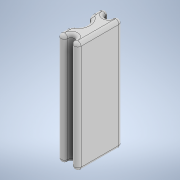
# Autodesk Inventor part: CableBase
Saved by Autodesk Inventor 2020 (Build 240168000, 168)
## iProperties
Created: 2020-07-28
Part Number: CableBase
Material: Generic
Document SubType Name: Modeling
Designer: maple
Density: 1 g/cm^3
Appearance: Default
Author: maple
Autodesk Inventor part; units mm, degrees
ref_plane "YZ Plane" through (0, 0, 0) normal (1, 0, 0) x (0, 1, 0)
ref_plane "XZ Plane" through (0, 0, 0) normal (0, 1, 0) x (-1, 0, 0)
ref_plane "XY Plane" through (0, 0, 0) normal (0, 0, 1) x (1, 0, 0)
sketch "Sketch1" plane through (0, 0, 0) normal (0, 1, 0) x (-1, 0, 0)
  line L0 (0, 0) -> (3, 0)
  line L1 (3, 0) -> (3, -20)
  line L2 (3, -20) -> (0, -20)
  line L3 (0, -20) -> (0, 0)
  line L4 (3, 0) -> (6, 0)
  line L5 (6, 0) -> (6, -3)
  line L6 (6, -3) -> (3, -3)
  line L7 (3, -3) -> (3, 0)
  line L8 (3, -20) -> (6, -20)
  line L9 (6, -20) -> (6, -17)
  line L10 (6, -17) -> (3, -17)
  line L11 (3, -17) -> (3, -20)
  line L12 (3, -3) -> (9, -3)
  line L13 (9, -3) -> (9, -6)
  line L14 (9, -6) -> (3, -6)
  line L15 (3, -6) -> (3, -3)
  line L16 (3, -17) -> (9, -17)
  line L17 (9, -17) -> (9, -14)
  line L18 (9, -14) -> (3, -14)
  line L19 (3, -14) -> (3, -17)
  line L20 (9, -17) -> (6, -17)
  line L21 (6, -17) -> (6, -20)
  line L22 (6, -20) -> (9, -20)
  line L23 (9, -20) -> (9, -17)
  line L24 (9, -3) -> (6, -3)
  line L25 (6, -3) -> (6, 0)
  line L26 (6, 0) -> (9, 0)
  line L27 (9, 0) -> (9, -3)
  line L28 (6, -6) -> (6, -17)
  arc A0 (9, -6) -> (9, -14) centre (10.1667, -10) ccw
  dimension "d0" = 3
  dimension "d1" = 20
  dimension "d2" = 3
  dimension "d3" = 3
  dimension "d4" = 3
  dimension "d5" = 3
  dimension "d6" = 6
  dimension "d7" = 3
  dimension "d8" = 6
  dimension "d9" = 3
  constraints: 58 end point, 14 parallel, 7 horizontal, 7 perpendicular, 2 point on circle, 1 centre point, 1 midpoint, 1 tangent
  measures "d0" distance of L1.end L2.end
  measures "d1" distance of L0.end L1.end
  measures "d2" distance of L5.end L6.end
  measures "d3" distance of L4.end L5.end
  measures "d4" distance of L10.end L9.end
  measures "d5" distance of L9.end L8.end
  measures "d6" distance of L13.end L14.end
  measures "d7" distance of L12.end L13.end
  measures "d8" distance of L18.end L17.end
  measures "d9" distance of L17.end L16.end
extrude "Extrusion1" add sketch "Sketch1" along normal blind 50 contours L0 L1 L2 L3 | L6 L12 L13 L14 L1 | L26 L27 L12 L5 | L14 L28 L18 L1 | L1 L18 L28 L10 | L9 L16 L23 L22 | L14 A0 L28 | L28 L18 L17 L16 | L28 A0 L18
fillet "Fillet1" radius 1.5 12 edges at (-9, 25, -20) (-6, 25, -20) (-6, 25, -17) (-3, 25, -20) (-3, 25, -17) (0, 25, -20) (-9, 25, 0) (-6, 25, 0) (-6, 25, -3) (-3, 25, -3) (-3, 25, 0) (0, 25, 0)
fillet "Fillet2" radius 3 2 edges at (-9, 25, -14) (-9, 25, -6)
fillet "Fillet3" radius 1.5 40 edges at (-8.5607, 0, -19.5607) (-7.5, 0, -20) (-9, 0, -16.4155) (-8.6676, 0, -14.4585) (-6, 0, -10) (-8.6676, 0, -5.5415) (-9, 0, -3.5845) (-8.5607, 0, -0.4393) (-7.5, 0, 0) (-6, 0, -1.5) (-4.5, 0, -3) (-3, 0, -1.5) (-2.5607, 0, -0.4393) (-1.5, 0, 0) (0, 0, -10) (-3, 0, -18.5) (-2.5607, 0, -19.5607) (-1.5, 0, -20) (-6, 0, -18.5) (-4.5, 0, -17) (-8.6676, 50, -5.5415) (-9, 50, -3.5845) (-8.5607, 50, -0.4393) (-7.5, 50, 0) (-6, 50, -1.5) (-4.5, 50, -3) (-3, 50, -1.5) (-2.5607, 50, -0.4393) (-1.5, 50, 0) (0, 50, -10) (-3, 50, -18.5) (-2.5607, 50, -19.5607) (-1.5, 50, -20) (-6, 50, -18.5) (-4.5, 50, -17) (-8.5607, 50, -19.5607) (-7.5, 50, -20) (-9, 50, -16.4155) (-8.6676, 50, -14.4585) (-6, 50, -10)
body "Solid1"
